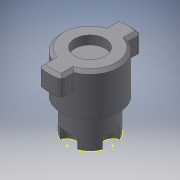
# Autodesk Inventor part: conecter
Saved by Autodesk Inventor 2018 (Build 220112000, 112)
## iProperties
Created: 2019-02-27
Part Number: conecter
Material: 一般
Document SubType Name: Modeling
Designer: ku_sk
Density: 1 g/cm^3
Appearance: 既定
Author: ku_sk
## iProperties of the stored document conecter_3D プリント.ipt
Created: 2019-03-14
Part Number: conecter_3D プリント
Material: 一般
Document SubType Name: Modeling
Designer: ku_sk
Density: 1 g/cm^3
Appearance: 既定
Author: ku_sk
Autodesk Inventor part; units mm, degrees
ref_plane "YZ Plane" through (0, 0, 0) normal (1, 0, 0) x (0, 1, 0)
ref_plane "XZ Plane" through (0, 0, 0) normal (0, 1, 0) x (-1, 0, 0)
ref_plane "XY Plane" through (0, 0, 0) normal (0, 0, 1) x (1, 0, 0)
sketch "スケッチ1" plane through (0, 0, 0) normal (0, 0, 1) x (1, 0, 0)
  circle A0 centre (0, 0) radius 10
  dimension "d0" = 20
  constraints: 1 centre point, 1 coincident
  measures "d0" diameter of A0
extrude "押し出し1" add sketch "スケッチ1" along normal blind 6.5
sketch "スケッチ2" plane through (0, 0, 0) normal (0, 0, -1) x (-1, 0, 0)
  arc A0 (3.75, 13.4884) -> (-3.75, 13.4884) centre (0, 0) ccw
  arc A1 (-3.75, -13.4884) -> (3.75, -13.4884) centre (0, 0) ccw
  circle A2 centre (0, 0) radius 10 projected
  line L0 (-3.75, 13.4884) -> (-3.75, -13.4884)
  line L1 (3.75, -13.4884) -> (3.75, 13.4884)
  line L2 (0, -19.6) -> (0, 19.6) projected
  line L3 (14, 0) -> (-14, 0) projected
  point P0 (0, 14)
  point P1 (0, -14)
  point P2 (-3.75, 0)
  dimension "d3" = 14
  dimension "d4" = 7.5
  constraints: 6 point on circle, 4 end point, 3 point on line, 2 centre point, 2 concentric, 1 midpoint, 1 parallel
  measures "d3" radius of A0
  measures "d4" distance between parallel lines of L1 L0
extrude "押し出し2" add sketch "スケッチ2" against normal up to surface (6.5 mm away) contours L1 A2 L2 A0 | L2 A2 L0 A0 | L1 L3 L2 A2 | L2 L3 L0 A2 | L1 A2 L2 L3 | L2 A2 L0 L3 | L1 A1 L2 A2 | L2 A1 L0 A2
chamfer "面取り1" distance 1 angle 45 8 edges at (-10, 0, 6.5) (10, 0, 6.5) (-3.75, 11.3793, 6.5) (0, 14, 6.5) (3.75, 11.3793, 6.5) (3.75, -11.3793, 6.5) (0, -14, 6.5) (-3.75, -11.3793, 6.5)
fillet "フィレット1" radius 1 4 edges at (-3.75, -13.4884, 2.75) (3.75, -13.4884, 2.75) (3.75, 13.4884, 2.75) (-3.75, 13.4884, 2.75)
sketch "スケッチ4" plane through (0, 0, 0) normal (0, 0, -1) x (-1, 0, 0)
  circle A0 centre (0, 0) radius 8
  dimension "d14" = 16
  constraints: 1 centre point, 1 coincident
  measures "d14" diameter of A0
extrude "押し出し4" add sketch "スケッチ4" along normal blind 19
sketch "スケッチ5" plane through (0, 0, 6.5) normal (0, 0, 1) x (1, 0, 0)
  circle A0 centre (0, 0) radius 5.25
  dimension "d17" = 10.5
  constraints: 1 centre point, 1 coincident
  measures "d17" diameter of A0
extrude "押し出し5" cut sketch "スケッチ5" against normal blind 3
sketch "スケッチ6" plane through (0, 0, -19) normal (0, 0, -1) x (-1, 0, 0)
  circle A0 centre (0, 7.85) radius 3.05
  line L0 (14, 0) -> (-14, 0) projected
  line L1 (0, -19.6) -> (0, 19.6) projected
  point P0 (0, 0)
  dimension "d20" = 6.1
  dimension "d21" = 7.85
  constraints: 1 centre point, 1 point on line
  measures "d20" diameter of A0
  measures "d21" distance of point (0, 0) A0.centre
extrude "押し出し6" cut sketch "スケッチ6" against normal blind 4
pattern_circular "円形状パターン1" count 4 over 360 about axis through (0, 0, -10) along (0, 0, 1) of "押し出し6"
sketch "スケッチ7" plane through (0, 0, 0) normal (0, 0, -1) x (-1, 0, 0)
  circle A0 centre (0, 0) radius 5.25 projected
  circle A1 centre (0, 0) radius 10
  point P0 (-3.75, -9.2702)
  constraints: 1 coincident, 3 other
extrude "押し出し7" add sketch "スケッチ7" along normal blind 8
sketch "スケッチ8" plane through (0, 0, -19) normal (0, 0, -1) x (-1, 0, 0)
  arc A0 (-7.4089, -3.0179) -> (-7.4089, 3.0179) centre (-7.85, 0) ccw projected
  arc A1 (-7.4089, -3.0179) -> (-3.0179, -7.4089) centre (0, 0) ccw projected
  arc A2 (3.0179, -7.4089) -> (-3.0179, -7.4089) centre (0, -7.85) ccw projected
  arc A3 (3.0179, -7.4089) -> (7.4089, -3.0179) centre (0, 0) ccw projected
  arc A4 (7.4089, 3.0179) -> (7.4089, -3.0179) centre (7.85, 0) ccw projected
  arc A5 (7.4089, 3.0179) -> (3.0179, 7.4089) centre (0, 0) ccw projected
  arc A6 (-3.0179, 7.4089) -> (3.0179, 7.4089) centre (0, 7.85) ccw projected
  arc A7 (-3.0179, 7.4089) -> (-7.4089, 3.0179) centre (0, 0) ccw projected
extrude "押し出し8" add sketch "スケッチ8" along normal blind 0.708
